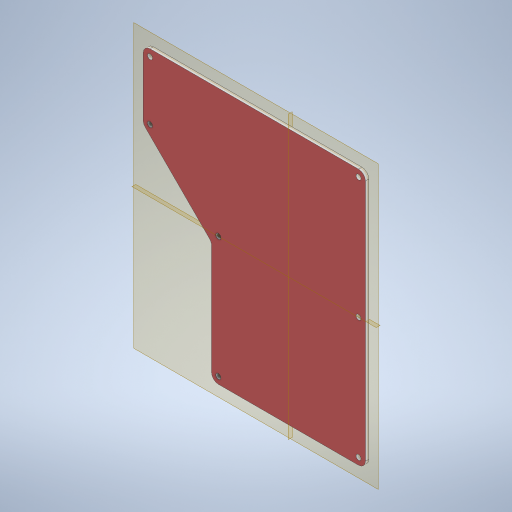
# Autodesk Inventor part: Контур платы
Saved by Autodesk Inventor 2023.2 (Build 272271030, 271C)
## iProperties
Created: 2024-03-22
Part Number: Контур платы
Material: Типовые
Document SubType Name: Modeling
Designer: I9232
Density: 1 g/cm^3
Appearance: По умолчанию
Author: I9232
Autodesk Inventor part; units mm, degrees
sketch "Эскиз1" plane through (0, 0, 0) normal (0, 0, 1) x (1, 0, 0)
  line L0 (-45, -75) -> (45, -75)
  line L1 (45, -75) -> (45, 75)
  line L2 (45, 75) -> (-85, 75)
  line L3 (-45, 0) -> (-45, -75)
  line L4 (-45, -75) -> (45, 75) construction
  line L5 (45, -75) -> (-45, 75) construction
  line L6 (-85, 75) -> (-85, 0)
  line L7 (-85, 0) -> (-49.5, 0)
  line L8 (-45, 0) -> (-85, 0)
  line L9 (-45, -5) -> (-85, 35)
  point P0 (0, 0)
  dimension "d0" = 90
  dimension "d1" = 150
  dimension "d22" = 75
  dimension "d25" = 130
  dimension "d26" = 45
  dimension "d27" = 40
  constraints: 20 end point, 3 perpendicular, 3 point on line, 2 midpoint, 2 parallel, 1 collinear, 1 horizontal
  measures "d0" distance of L0.start L0.end
  measures "d1" distance of L0.end L1.end
  measures "d22" distance of L2.end L6.end
  measures "d25" distance of L1.end L2.end
  measures "d26" angle of L3 L9
  measures "d27" distance of L9.end L2.end
extrude "Выдавливание1" add sketch "Эскиз1" along normal mid plane 2 contours L3 L8 L7 L9 L6 L2 L1 L0 | L9 L7 L8 L3
fillet "Сопряжение2" radius 4 6 edges at (45, 75, 0) (45, -75, 0) (-45, -75, 0) (-45, -5, 0) (-85, 35, 0) (-85, 75, 0)
sketch "Эскиз4" plane through (0, 0, 1) normal (0, 0, 1) x (1, 0, 0)
  circle A0 centre (-81, 36.6569) radius 1.5
  circle A1 centre (-41, 0) radius 1.5
  circle A2 centre (41, 0) radius 1.5
  circle A3 centre (41, -71) radius 1.5
  circle A4 centre (-41, -71) radius 1.5
  circle A5 centre (41, 71) radius 1.5
  circle A6 centre (-81, 71) radius 1.5
  arc A7 (-81, 75) -> (-85, 71) centre (-81, 71) ccw construction
  line L0 (-85, 71) -> (-85, 36.6569) construction
  arc A8 (-85, 36.6569) -> (-83.8284, 33.8284) centre (-81, 36.6569) ccw construction
  line L1 (-83.8284, 33.8284) -> (-46.1716, -3.8284) construction
  arc A9 (-45, -6.6569) -> (-46.1716, -3.8284) centre (-49, -6.6569) ccw construction
  line L2 (-45, -6.6569) -> (-45, -71) construction
  arc A10 (-45, -71) -> (-41, -75) centre (-41, -71) ccw construction
  line L3 (-41, -75) -> (41, -75) construction
  arc A11 (41, -75) -> (45, -71) centre (41, -71) ccw construction
  line L4 (45, -71) -> (45, 71) construction
  arc A12 (45, 71) -> (41, 75) centre (41, 71) ccw construction
  line L5 (41, 75) -> (-81, 75) construction
  line L6 (-81, 71) -> (-81, 36.6569) construction
  line L7 (-81, 36.6569) -> (-43.3431, -1) construction
  arc A13 (-41, -6.6569) -> (-43.3431, -1) centre (-49, -6.6569) ccw construction
  line L8 (-41, -6.6569) -> (-41, -71) construction
  line L9 (-41, -71) -> (41, -71) construction
  line L10 (41, -71) -> (41, 71) construction
  line L11 (41, 71) -> (-81, 71) construction
  line L12 (-112.1598, 0) -> (72.1598, 0) projected
  point P0 (0, 0)
  point P1 (41, 0)
  dimension "d29" = 3
  dimension "d30" = 4
  dimension "d31" = 41
  constraints: 12 end point, 8 centre point, 6 coincident, 6 equal radius, 2 point on circle, 1 midpoint, 1 point on line, 6 other
  measures "d29" diameter of A0
  measures "d30" distance between parallel lines of L0 L6
  measures "d31" distance of point (0, 0) A1.centre
extrude "Выдавливание4" cut sketch "Эскиз4" against normal through all
